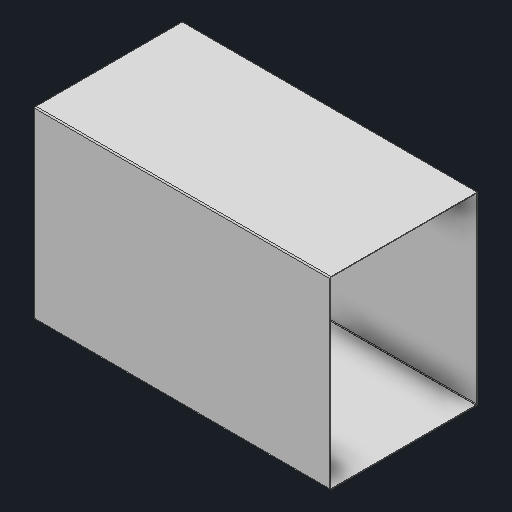
# Autodesk Inventor part: Reflector
Saved by Autodesk Inventor 2026.1 (Build 301233000, 233)
## iProperties
Created: 2026-07-13
Part Number: Reflector
Material: Generic
Document SubType Name: Sheet Metal
Designer: aleja
Density: 1 g/cm^3
Sheet Metal Rule: Default_mm
Appearance: Default
Author: aleja
Autodesk Inventor part; units mm, degrees
ref_plane "YZ Plane" through (0, 0, 0) normal (1, 0, 0) x (0, 1, 0)
ref_plane "XZ Plane" through (0, 0, 0) normal (0, 1, 0) x (-1, 0, 0)
ref_plane "XY Plane" through (0, 0, 0) normal (0, 0, 1) x (1, 0, 0)
sketch "Sketch1" plane through (0, 0, 0) normal (0, 1, 0) x (-1, 0, 0)
  line L0 (-120, 75) -> (120, 75)
  line L1 (120, 75) -> (120, -75)
  line L2 (120, -75) -> (-120, -75)
  line L3 (-120, -75) -> (-120, 75)
  line L4 (-120, 75) -> (120, -75) construction
  line L5 (120, 75) -> (-120, -75) construction
  point P0 (0, 0)
  dimension "d0" = 150
  dimension "d1" = 240
  measures "d0" distance of L0.end L1.end
  measures "d1" distance of L1.end L2.end
extrude "Plate1" add sketch "Sketch1" along normal blind 0.5
sketch "Sketch4" plane through (120, 0, 74.5) normal (0, 0, 1) x (1, 0, 0)
  line L0 (-240, 0) -> (0, 0)
  line L1 (0, 0) -> (0, 120)
  line L2 (0, 120) -> (-240, 120)
  line L3 (-240, 120) -> (-240, 0)
  constraints: 6 end point, 1 horizontal, 1 perpendicular, 1 vertical
edge flange "Flange1" height 120 angle 90 thickness 0.5 bend radius 0.5 thickness toward (0, 0, 1) relief tear relief width 0.5 relief depth 0.25 edges at (0, 0.5, 75) wall of the first edge with corners at (-120, 0, 74.5) (120, 0, 74.5) (120, 120, 74.5) (-120, 120, 74.5)
bend "Bend1"
corner "Corner1"
sketch "Sketch5" plane through (-120, 0, -74.5) normal (0, 0, -1) x (-1, 0, 0)
  line L0 (-240, 0) -> (0, 0)
  line L1 (0, 0) -> (0, 120)
  line L2 (0, 120) -> (-240, 120)
  line L3 (-240, 120) -> (-240, 0)
  constraints: 6 end point, 1 horizontal, 1 perpendicular, 1 vertical
edge flange "Flange2" height 120 angle 90 thickness 0.5 bend radius 0.5 thickness toward (0, 0, -1) relief tear relief width 0.5 relief depth 0.25 edges at (0, 0.5, -75) wall of the first edge with corners at (120, 0, -74.5) (-120, 0, -74.5) (-120, 120, -74.5) (120, 120, -74.5)
bend "Bend2"
corner "Corner2"
sketch "Sketch6" plane through (-120, 119.5, -75) normal (0, 1, 0) x (-1, 0, 0)
  line L0 (-240, 0) -> (0, 0)
  line L1 (0, 0) -> (0, 149)
  line L2 (0, 149) -> (-240, 149)
  line L3 (-240, 149) -> (-240, 0)
  constraints: 6 end point, 1 horizontal, 1 perpendicular, 1 vertical
edge flange "Flange3" height 149 angle 90 thickness 0.5 bend radius 0.5 thickness toward (0, 1, 0) relief tear relief width 0.5 relief depth 0.25 edges at (0, 120, -74.5) wall of the first edge with corners at (120, 119.5, -75) (-120, 119.5, -75) (-120, 119.5, 74) (120, 119.5, 74)
bend "Bend3"
corner "Corner3"
equation "\"d2\" = Thickness"
equation "\"d12\" = BendReliefWidth"
equation "\"d13\" = BendReliefDepth"
equation "\"d14\" = MinimumRemnant"
equation "\"d15\" = TransitionRadius"
equation "\"d18\" = BendRadius"
equation "\"d19\" = CornerReliefSize"
equation "\"d20\" = GapSize"
equation "\"d21\" = JacobiRadiusSize"
equation "\"d22\" = BendReliefWidth"
equation "\"d23\" = BendReliefDepth"
equation "\"d24\" = MinimumRemnant"
equation "\"d25\" = TransitionRadius"
equation "\"d28\" = BendRadius"
equation "\"d29\" = CornerReliefSize"
equation "\"d30\" = GapSize"
equation "\"d31\" = JacobiRadiusSize"
equation "\"d32\" = BendReliefWidth"
equation "\"d33\" = BendReliefDepth"
equation "\"d34\" = MinimumRemnant"
equation "\"d35\" = TransitionRadius"
equation "\"d38\" = BendRadius"
equation "\"d39\" = CornerReliefSize"
equation "\"d40\" = GapSize"
equation "\"d41\" = JacobiRadiusSize"
equation "\"BendRadius\" = Thickness"
equation "\"BendReliefWidth\" = Thickness"
equation "\"BendReliefDepth\" = 0.5 * Thickness"
equation "\"CornerReliefSize\" = 4 * Thickness"
equation "\"MinimumRemnant\" = 2 * Thickness"
equation "\"TransitionRadius\" = BendRadius"
equation "\"JacobiRadiusSize\" = BendRadius"
equation "\"GapSize\" = Thickness"
equation "\"Thickness\" = 0.5"
body "Solid1"
